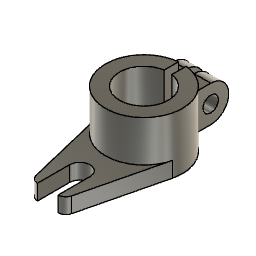
Part 2_ Basic 3D modeling v1 (Autodesk Fusion 360 design; units mm, degrees)
Autodesk Fusion 360 part; units mm, degrees
cylinder "CylinderPrimitive1" add diameter 60 height 44 placed x (1, 0, 0) y (0, 1, 0) z (0, 0, 1) at (0, 0, 0)
cylinder "CylinderPrimitive2" cut diameter 38 height 44 placed x (1, 0, 0) y (0, 1, 0) z (0, 0, 1) at (0, 0, 0)
sketch "Sketch3" plane through (0, 0, 0) normal (0, 0, 1) x (1, 0, 0)
  line L0 (7.9986, -49.8503) -> (7.9986, -74.8503)
  line L1 (7.9986, -49.8503) -> (7.9986, -74.8503)
  line L2 (-7.9986, -49.8503) -> (-7.9986, -74.8503)
  line L3 (-29.1548, -7.0708) -> (-13.8286, -70.2644)
  circle A0 centre (0, 0) radius 30
  line L4 (29.1548, -7.0708) -> (13.8286, -70.2644)
  arc A1 (7.9986, -50.1497) -> (-7.9986, -50.1497) centre (0, -50) ccw
  arc A2 (-13.8286, -70.2644) -> (-7.9986, -74.8503) centre (-7.9977, -68.8503) ccw
  arc A3 (7.9986, -74.8503) -> (13.853, -70.1639) centre (7.9986, -68.8503) ccw
  dimension "d5" = 50
  dimension "d6" = 16
  dimension "d8" = 25
  dimension "d9" = 25
  dimension "d10" = 25
  dimension "d11" = 12
  dimension "d12" = 12
  constraint coincident L2.start A1
  constraint coincident L0.start A1
  constraint tangent L3 A2
  constraint tangent L3 A0
  constraint coincident L3.start A0
  constraint coincident L2 A1.end
  constraint coincident L0 A1.start
  constraint coincident L4 A3.end
  measures "d5" distance of A0.centre A1.centre
  measures "d6" diameter of A1
  measures "d8" distance of L0.start L0.end
  measures "d9" distance of L0.start L0.end
  measures "d10" distance of L2.start L2.end
  measures "d11" diameter of A2
  measures "d12" diameter of A3
extrude "Extrude1" add sketch "Sketch3" along normal blind 12 contours L0 L1 L2 L3 A0 L4 A1 A2 A3
sketch "Sketch4" plane through (0, 0, 0) normal (1, 0, 0) x (0, 1, 0)
  circle A0 centre (36, 22) radius 6
  arc A1 (36, 8) -> (36, 36) centre (36, 22) ccw
  line L0 (36, 36) -> (0, 36)
  line L1 (0, 36) -> (0, 8)
  line L2 (0, 8) -> (36, 8)
  dimension "d17" = 28
  constraint tangent A1 L0
  constraint horizontal L0
  constraint perpendicular L0 L1
  constraint tangent A1 L2
  measures "d17" diameter of A1
extrude "Extrude2" add sketch "Sketch4" along normal blind 13 from surface at 3
move_face "OffsetFaces1" offset 16 1 faces at (3, 33.5048, 10.7168)
extrude "Extrude3" cut sketch "Sketch4" along normal mid plane 6
cylinder "CylinderPrimitive3" cut diameter 38 height 44 placed x (1, 0, 0) y (0, 1, 0) z (0, 0, 1) at (0, 0, 0)
sketch "Sketch6" plane through (0, 0, 0) normal (0, 0, 1) x (1, 0, 0)
  line L0 (-3, 18.7617) -> (-3, 29.8496)
  line L1 (3, 18.7617) -> (3, 29.8496)
  arc A0 (3, 29.8496) -> (-3, 29.8496) centre (0, 0) ccw
  arc A1 (3, 18.7617) -> (-3, 18.7617) centre (0, 0) ccw
  dimension "d29" = 60
  dimension "d30" = 38
  constraint coincident A0.centre A1.centre
  measures "d29" diameter of A0
  measures "d30" diameter of A1
extrude "Extrude4" cut sketch "Sketch6" along normal blind 44
